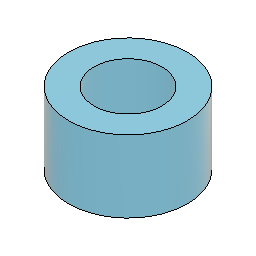
M6 Screw Spacer v3 (Autodesk Fusion 360 design; units mm, degrees)
Autodesk Fusion 360 part; units mm, degrees
note: some values were not read from the file. Chosen so that the rebuilt part matches the saved one: which face or edge a step refers to.
cylinder "CylinderPrimitive1" add diameter 10 height 6.5 placed x (1, 0, 0) y (0, 0, -1) z (0, 1, 0) at (-3.244, 0, 0) makes body 1
move_body "Move1" bodies 1 to x (1, 0, 0) y (0, 1, 0) z (0, 0, 1) at (3, 0, 0)
move_body "Move2" bodies 1 to x (1, 0, 0) y (0, 1, 0) z (0, 0, 1) at (1, 0, 0)
move_body "Move3" bodies 1 to x (1, 0, 0) y (0, 1, 0) z (0, 0, 1) at (-0.756, 0, 0)
cylinder "CylinderPrimitive3" cut diameter 6 height -40 placed x (1, 0, 0) y (0, 0, -1) z (0, 1, 0) at (0, 6.5, 0) bodies 1
cylinder "CylinderPrimitive4" cut diameter 8 height -100 placed x (1, 0, 0) y (0, 0, -1) z (0, 1, 0) at (0, 6.5, 0) bodies 1
cylinder "CylinderPrimitive5" add diameter 14 height -6.5 placed x (1, 0, 0) y (0, 0, -1) z (0, 1, 0) at (0, 6.5, 0) bodies 1
cylinder "CylinderPrimitive6" cut diameter 8 height -25 placed x (1, 0, 0) y (0, 0, -1) z (0, 1, 0) at (0, 6.5, 0) bodies 1
extrude "Extrude1" add 1 faces at (5.9739, 6.5, 0.3478) along direction (0, 1, 0) blind 2 on bodies 1 bodies 1
copy_body "Body->Comp1" bodies 1 removing the originals makes body 2 in component "M6 Spacer"
component "M6 Spacer" placed x (1, 0, 0) y (0, 1, 0) z (0, 0, 1) at (0, 0, 0)
